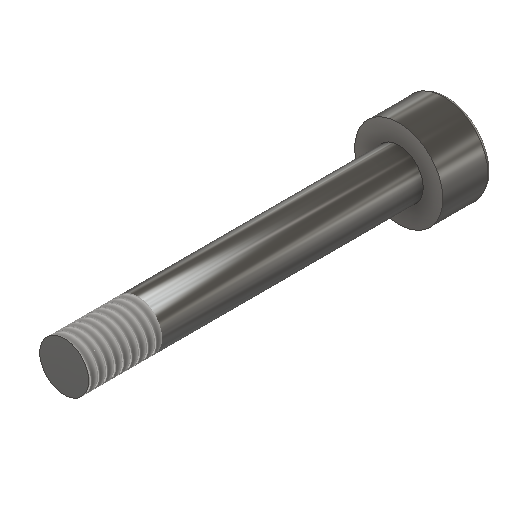
# Autodesk Inventor part: COTS_GENERIC_Solenoid_Actuator_Push_Rod_M3
Saved by Autodesk Inventor 2026.1 (Build 301233000, 233)
## iProperties
Created: 2018-06-14
Part Number: COTS_GENERIC_Solenoid_Actuator_Push_Rod_M3
Material: Generic
Document SubType Name: Modeling
Designer: Andrzej
Density: 1 g/cm^3
Appearance: Steel - Polished
Author: Andrzej
Autodesk Inventor part; units mm, degrees
ref_plane "YZ Plane" through (0, 0, 0) normal (1, 0, 0) x (0, 1, 0)
ref_plane "XZ Plane" through (0, 0, 0) normal (0, 1, 0) x (-1, 0, 0)
ref_plane "XY Plane" through (0, 0, 0) normal (0, 0, 1) x (1, 0, 0)
sketch "Sketch1" plane through (0, 0, 0) normal (0, 0, 1) x (1, 0, 0)
  circle A0 centre (0, 0) radius 1.5
  circle A1 centre (0, 0) radius 2.7
  dimension "d0" = 3
  dimension "d5" = 5.4
  constraints: 2 centre point, 2 coincident
  measures "d0" diameter of A0
  measures "d5" diameter of A1
extrude "Extrusion1" add sketch "Sketch1" along normal blind 20.5 contours A0
extrude "Extrusion2" add sketch "Sketch1" against normal blind 3 contours A0 | A1
thread "Thread2" size "M3x0.5" class "6g" standard "ANSI Metric M Profile" length 4.5
fillet "Fillet1" radius 0.25 1 edges at (-2.7, 0, -3)
sketch "Sketch2" plane through (0, 0, -3) normal (0, 0, -1) x (-1, 0, 0)
  circle A0 centre (0, 0) radius 1.5 projected
  line L0 (-1.5, 0) -> (-0.75, 1.299)
  line L1 (-0.75, 1.299) -> (0.75, 1.299)
  line L2 (0.75, 1.299) -> (1.5, 0)
  line L3 (1.5, 0) -> (0.75, -1.299)
  line L4 (0.75, -1.299) -> (-0.75, -1.299)
  line L5 (-0.75, -1.299) -> (-1.5, 0)
  constraints: 12 end point, 1 coincident, 1 horizontal alignment, 14 other
extrude "Extrusion3" cut sketch "Sketch2" against normal blind 2 contours L3 L4 L5 L0 L1 L2
body "Solid1"
